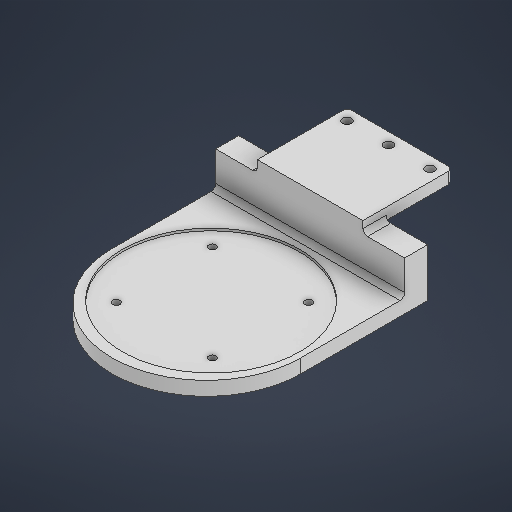
# Autodesk Inventor part: lidar base
Saved by Autodesk Inventor 2026.2 (Build 302298000, 298)
## iProperties
Created: 2025-12-10
Part Number: lidar base
Material: 一般
Document SubType Name: Modeling
Designer: user
Density: 1 g/cm^3
Appearance: 預設
Author: user
Autodesk Inventor part; units mm, degrees
ref_plane "YZ Plane" through (0, 0, 0) normal (1, 0, 0) x (0, 1, 0)
ref_plane "XZ Plane" through (0, 0, 0) normal (0, 1, 0) x (-1, 0, 0)
sketch "草圖1" plane through (0, 0, 0) normal (0, 1, 0) x (-1, 0, 0)
  line L0 (22.9, 7.0791) -> (-22.9, 7.0791)
  line L1 (-22.9, 7.0791) -> (-22.9, -19.9209)
  line L2 (-20.9, -21.9209) -> (20.9, -21.9209)
  line L3 (22.9, -19.9209) -> (22.9, 7.0791)
  arc A0 (20.9, -21.9209) -> (22.9, -19.9209) centre (20.9, -19.9209) ccw
  arc A1 (-22.9, -19.9209) -> (-20.9, -21.9209) centre (-20.9, -19.9209) ccw
  line L4 (0, -28.2179) -> (0, 12.962) projected
  circle A2 centre (0, -16.9209) radius 2
  circle A3 centre (-18, -16.9209) radius 2
  circle A4 centre (18, -16.9209) radius 2
  point P0 (0, 0)
  dimension "d2" = 2
  dimension "d3" = 4
  dimension "d4" = 18
  dimension "d5" = 4
  dimension "d6" = 24
  dimension "d9" = 5
  constraints: 8 end point, 5 centre point, 4 point on circle, 4 tangent, 2 parallel, 1 equal radius, 1 horizontal, 1 perpendicular, 1 point on line, 1 symmetric about line, 2 other
  measures "d2" radius of A0
  measures "d3" diameter of A2
  measures "d4" distance of A3.centre A2.centre
  measures "d5" diameter of A3
  measures "d6" distance from line of L0 A2.centre
  measures "d9" distance from line of L2 A2.centre
extrude "擠出1" add sketch "草圖1" along normal mid plane 5 contours L3 A0 L2 L4 A2 L0 | L4 A2 L2 A1 L1 L0
sketch "草圖3" plane through (-22.9, 2.5, 7.0791) normal (0, 0, 1) x (1, 0, 0)
  line L0 (0, -5) -> (0, 0) projected
  line L1 (0, 0) -> (45.8, 0) projected
  line L2 (45.8, -5) -> (45.8, 0) projected
  line L3 (0, 0) -> (45.8, 0)
  line L4 (45.8, 0) -> (45.8, -5)
  line L5 (0, -5) -> (0, 0)
  line L6 (0, 0) -> (45.8, -5) construction
  line L7 (45.8, 0) -> (0, -5) construction
  line L8 (24.9, -5) -> (20.9, -5) projected
  line L9 (-18.1, -5) -> (63.9, -5)
  line L10 (-18.1, -5) -> (-18.1, -28)
  line L11 (-18.1, -28) -> (63.9, -28)
  line L12 (63.9, -28) -> (63.9, -5)
  point P0 (22.9, -2.5)
  point P1 (22.9, -5)
  dimension "d12" = 82
  dimension "d13" = 23
  constraints: 18 end point, 4 midpoint, 3 perpendicular, 2 horizontal, 1 parallel, 1 vertical
  measures "d12" distance of L9.start L9.end
  measures "d13" distance of L9.start L10.end
extrude "擠出2" add sketch "草圖3" along normal blind 10
ref_plane "工作平面1" through (0, -17.5, 0) normal (0, 1, 0) x (1, 0, 0)
sketch "草圖5" plane through (0, -17.5, 0) normal (0, 1, 0) x (1, 0, 0)
  line L0 (-41, -17.0791) -> (41, -17.0791) projected
  line L1 (-41, -17.0791) -> (41, -17.0791)
  line L2 (41, -17.0791) -> (41, -62.0791)
  line L3 (0, -103.0791) -> (0, -103.0791)
  line L4 (-41, -62.0791) -> (-41, -17.0791)
  arc A0 (0, -103.0791) -> (41, -62.0791) centre (0, -62.0791) ccw
  arc A1 (-41, -62.0791) -> (0, -103.0791) centre (0, -62.0791) ccw
  point P0 (0, 0)
  point P1 (41, -103.0791)
  point P2 (-41, -103.0791)
  point P3 (41, -17.0791)
  point P4 (0, -103.0791)
  dimension "d19" = 86
  dimension "d22" = 41
  dimension "d23" = 41
  dimension "d37" = 82
  constraints: 8 end point, 4 point on circle, 4 point on line, 4 tangent, 2 centre point, 2 parallel, 1 horizontal, 1 perpendicular
  measures "d19" distance of L1.end point (41, -103.079)
  measures "d22" radius of A0
  measures "d23" radius of A1
  measures "d37" distance between parallel lines of L2 L4
extrude "擠出3" add sketch "草圖5" against normal up to surface (8 mm away)
sketch "草圖6" plane through (0, -17.5, 0) normal (0, 1, 0) x (1, 0, 0)
  arc A0 (-41, -62.0791) -> (41, -62.0791) centre (0, -62.0791) ccw projected
  circle A1 centre (0, -60.0791) radius 38.5
  line L0 (-41, -17.0791) -> (41, -17.0791) projected
  point P0 (0, 0)
  dimension "d24" = 77
  dimension "d28" = 43
  constraints: 1 centre point
  measures "d24" diameter of A1
  measures "d28" distance from line of L0 A1.centre
fillet "圓角2" radius 2 1 edges at (0, -17.5, 17.0791)
extrude "擠出5" cut sketch "草圖6" against normal blind 1
sketch "草圖8" plane through (0, -18.5, 60.0791) normal (0, 1, 0) x (1, 0, 0)
  circle A0 centre (-20.8595, 21.4584) radius 1.6
  circle A1 centre (0, 0) radius 38.5 projected
  line L0 (0, 107) -> (0, -68) projected
  circle A2 centre (20.8595, 21.4584) radius 1.6
  circle A3 centre (20.8595, -20.2606) radius 1.6
  circle A4 centre (-20.8595, -20.2606) radius 1.6
  point P0 (0, 60.0791)
  dimension "d32" = 3.2
  dimension "d33" = 41.719
  dimension "d38" = 41.719
  constraints: 4 centre point, 2 symmetric about line, 2 other
  measures "d32" diameter of A0
  measures "d33" distance of A2.centre A0.centre
  measures "d38" distance of A3.centre A2.centre
extrude "擠出6" cut sketch "草圖8" against normal through all contours A0 | A2 | A3 | A4
fillet "圓角3" radius 2 3 edges at (22.9, -2.5, 12.0791) (-22.9, -2.5, 12.0791) (0, -2.5, 7.0791)
sketch "草圖9" plane through (41, -25.5, 7.0791) normal (1, 0, 0) x (0, 0, -1)
  line L0 (-55, 0) -> (-96, 0) projected
  line L1 (0, 23) -> (0, 0) projected
  line L2 (-96, 0) -> (0, 0)
  line L3 (0, 0) -> (0, 2)
  line L4 (0, 2) -> (-96, 2)
  line L5 (-96, 2) -> (-96, 0)
  point P0 (7.0791, 25.5)
  dimension "d39" = 2
  constraints: 8 end point, 2 parallel, 1 horizontal, 1 perpendicular, 1 point on line
  measures "d39" distance of L4.end L0.end
extrude "擠出7" cut sketch "草圖9" against normal through all
